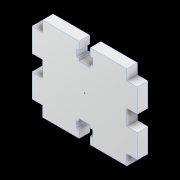
# Autodesk Inventor part: SmallSideFrame_04
Saved by Autodesk Inventor 2022 (Build 260153000, 153)
## iProperties
Created: 2021-03-08
Part Number: SmallSideFrame_04
Material: Aluminum 6061
Document SubType Name: Modeling
Designer: M3rob
Density: 2.7 g/cm^3
Appearance: Aluminum - Flat
Mass: 381.59 g
Surface Area: 298.895 cm^2
Volume: 141.33 cm^3
Author: M3rob
Autodesk Inventor part; units mm, degrees
ref_plane "YZ Plane" through (0, 0, 0) normal (1, 0, 0) x (0, 1, 0)
ref_plane "XZ Plane" through (0, 0, 0) normal (0, 1, 0) x (-1, 0, 0)
ref_plane "XY Plane" through (0, 0, 0) normal (0, 0, 1) x (1, 0, 0)
sketch "Sketch1" plane through (0, 0, 0) normal (0, 0, 1) x (1, 0, 0)
  line L0 (-50.8, 50.8) -> (-50.8, 38.1)
  line L1 (-50.8, -50.8) -> (-6.7437, -50.8)
  line L2 (50.8, -50.8) -> (50.8, -38.1)
  line L3 (50.8, 50.8) -> (6.7437, 50.8)
  line L4 (-50.8, 0) -> (50.8, 0) construction
  line L5 (-50.8, 38.1) -> (-63.5, 38.1)
  line L6 (-63.5, 38.1) -> (-63.5, 9.525)
  line L7 (-63.5, 9.525) -> (-50.8, 9.525)
  line L8 (-50.8, -9.525) -> (-63.5, -9.525)
  line L9 (-63.5, -9.525) -> (-63.5, -38.1)
  line L10 (-63.5, -38.1) -> (-50.8, -38.1)
  line L11 (50.8, 38.1) -> (63.5, 38.1)
  line L12 (63.5, 38.1) -> (63.5, 9.525)
  line L13 (63.5, 9.525) -> (50.8, 9.525)
  line L14 (50.8, -9.525) -> (63.5, -9.525)
  line L15 (63.5, -9.525) -> (63.5, -38.1)
  line L16 (63.5, -38.1) -> (50.8, -38.1)
  line L17 (-50.8, 38.1) -> (-50.8, 9.525) construction
  line L18 (-50.8, 9.525) -> (-50.8, -9.525)
  line L19 (-50.8, -9.525) -> (-50.8, -38.1) construction
  line L20 (-50.8, -38.1) -> (-50.8, -50.8)
  line L21 (50.8, -9.525) -> (50.8, 9.525)
  line L22 (50.8, -38.1) -> (50.8, -9.525) construction
  line L23 (50.8, 9.525) -> (50.8, 38.1) construction
  line L24 (50.8, 38.1) -> (50.8, 50.8)
  line L25 (-6.7437, 50.8) -> (-6.7437, 41.275)
  line L26 (-6.7437, 41.275) -> (-9.525, 41.275)
  line L27 (-9.525, 41.275) -> (-9.525, 33.3375)
  line L28 (-9.525, 33.3375) -> (-6.7437, 33.3375)
  line L29 (-6.7437, 33.3375) -> (-6.7437, 30.1625)
  line L30 (-6.7437, 30.1625) -> (6.7437, 30.1625)
  line L31 (6.7437, 30.1625) -> (6.7437, 33.3375)
  line L32 (6.7437, 33.3375) -> (9.525, 33.3375)
  line L33 (9.525, 33.3375) -> (9.525, 41.275)
  line L34 (9.525, 41.275) -> (6.7437, 41.275)
  line L35 (6.7437, 41.275) -> (6.7437, 50.8)
  line L36 (0, 50.8) -> (0, 0) construction
  line L37 (-6.7437, -50.8) -> (-6.7437, -41.275)
  line L38 (-6.7437, -41.275) -> (-9.525, -41.275)
  line L39 (-9.525, -41.275) -> (-9.525, -33.3375)
  line L40 (-9.525, -33.3375) -> (-6.7437, -33.3375)
  line L41 (-6.7437, -33.3375) -> (-6.7437, -30.1625)
  line L42 (-6.7437, -30.1625) -> (6.7437, -30.1625)
  line L43 (6.7437, -30.1625) -> (6.7437, -33.3375)
  line L44 (6.7437, -33.3375) -> (9.525, -33.3375)
  line L45 (9.525, -33.3375) -> (9.525, -41.275)
  line L46 (9.525, -41.275) -> (6.7437, -41.275)
  line L47 (6.7437, -50.8) -> (6.7437, -41.275)
  line L48 (0, 50.8) -> (-6.7437, 50.8) construction
  line L49 (-6.7437, 50.8) -> (-50.8, 50.8)
  line L50 (6.7437, 50.8) -> (0, 50.8) construction
  line L51 (6.7437, -50.8) -> (50.8, -50.8)
  line L52 (-6.7437, -50.8) -> (6.7437, -50.8) construction
  dimension "d0" = 101.6
  dimension "d1" = 101.6
  dimension "d2" = 19.05
  dimension "d3" = 12.7
  dimension "d4" = 12.7
  dimension "d5" = 9.525
  dimension "d6" = 13.4874
  dimension "d7" = 7.9375
  dimension "d8" = 3.175
  dimension "d9" = 19.05
  constraints: 106 end point, 100 perpendicular, 21 point on line, 9 symmetric about line, 7 horizontal, 6 equal length, 3 horizontal alignment, 3 midpoint, 2 vertical, 1 coincident, 1 parallel, 4 other
  measures "d0" distance of L3.start L0.start
  measures "d1" distance of L2.start L3.start
  measures "d2" distance between parallel lines of L8 L7
  measures "d3" distance between parallel lines of L3 L5
  measures "d4" distance of L0.end L5.end
  measures "d5" distance of L34.end L3.end
  measures "d6" distance between parallel lines of L25 L35
  measures "d7" distance of L32.end L33.end
  measures "d8" distance of L30.end L31.end
  measures "d9" distance between parallel lines of L33 L27
extrude "Extrusion1" add sketch "Sketch1" along normal mid plane 12.7
sketch "Sketch3" plane through (0, 0, 6.35) normal (0, 0, 1) x (1, 0, 0)
  point P0 (0, 0)
body "Solid1"
